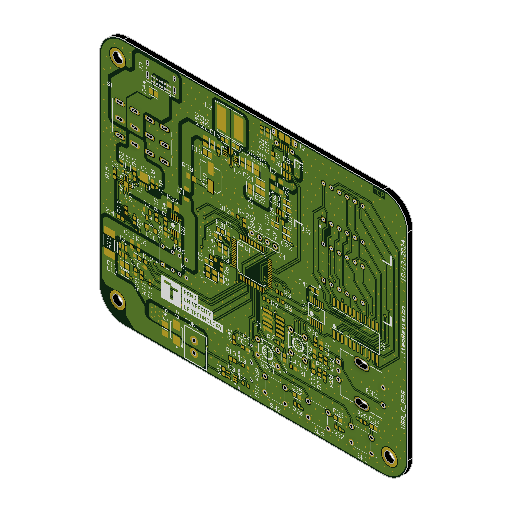
# Autodesk Inventor part: USB_C_PD_PPS_sink_BOARD
Saved by Autodesk Inventor 2025 (Build 290162000, 162)
## iProperties
Created: 2024-12-02
Part Number: USB_C_PD_PPS_sink_BOARD
Material: Generic
Document SubType Name: Modeling
Designer: Jan Mareš
Density: 1 g/cm^3
Appearance: BoardColor
Author: Jan Mareš
Autodesk Inventor part; units mm, degrees
ref_plane "YZ Plane" through (0, 0, 0) normal (1, 0, 0) x (0, 1, 0)
ref_plane "XZ Plane" through (0, 0, 0) normal (0, 1, 0) x (-1, 0, 0)
ref_plane "BoardFrontPlane" through (0, 0, 0) normal (0, 0, 1) x (1, 0, 0)
sketch "Sketch1" plane through (0, 0, 0) normal (0, 0, 1) x (1, 0, 0)
  arc A0 (0.0064, 8.0063) -> (8.0063, 0.0064) centre (8.0063, 8.0063) ccw
  line L0 (0.0064, 8.0063) -> (0.0064, 72.0063)
  arc A1 (8.0063, 80.0064) -> (0.0064, 72.0063) centre (8.0063, 72.0064) ccw
  line L1 (8.0063, 80.0064) -> (92.0063, 80.0064)
  arc A2 (100.0064, 72.0063) -> (92.0063, 80.0064) centre (92.0063, 72.0063) ccw
  line L2 (100.0064, 72.0063) -> (100.0064, 8.0063)
  arc A3 (92.0063, 0.0064) -> (100.0064, 8.0063) centre (92.0064, 8.0063) ccw
  line L3 (92.0063, 0.0064) -> (8.0063, 0.0064)
  constraints: 8 end point, 8 point on circle, 4 centre point
extrude "BoardOutline" add sketch "Sketch1" along normal blind 1.586
sketch "Sketch14" plane through (0, 0, 1.586) normal (0, 0, 1) x (1, 0, 0)
  point P0 (66.625, 25.884)
hole "S2-4" at (66.625, 25.884, 1.586) direction (0, 0, -1) diameter 1 end through all
sketch "Sketch15" plane through (0, 0, 1.586) normal (0, 0, 1) x (1, 0, 0)
  point P0 (66.625, 19.384)
hole "S2-3" at (66.625, 19.384, 1.586) direction (0, 0, -1) diameter 1 end through all
sketch "Sketch16" plane through (0, 0, 1.586) normal (0, 0, 1) x (1, 0, 0)
  point P0 (62.125, 25.884)
hole "S2-2" at (62.125, 25.884, 1.586) direction (0, 0, -1) diameter 1 end through all
sketch "Sketch17" plane through (0, 0, 1.586) normal (0, 0, 1) x (1, 0, 0)
  point P0 (62.125, 19.384)
hole "S2-1" at (62.125, 19.384, 1.586) direction (0, 0, -1) diameter 1 end through all
sketch "Sketch18" plane through (0, 0, 1.586) normal (0, 0, 1) x (1, 0, 0)
  point P0 (57.03, 46.534)
hole "J4-1" at (57.03, 46.534, 1.586) direction (0, 0, -1) diameter 1.02 end through all
sketch "Sketch19" plane through (0, 0, 1.586) normal (0, 0, 1) x (1, 0, 0)
  point P0 (49.41, 46.534)
hole "J4-4" at (49.41, 46.534, 1.586) direction (0, 0, -1) diameter 1.02 end through all
sketch "Sketch20" plane through (0, 0, 1.586) normal (0, 0, 1) x (1, 0, 0)
  point P0 (51.95, 46.534)
hole "J4-3" at (51.95, 46.534, 1.586) direction (0, 0, -1) diameter 1.02 end through all
sketch "Sketch21" plane through (0, 0, 1.586) normal (0, 0, 1) x (1, 0, 0)
  point P0 (54.49, 46.534)
hole "J4-2" at (54.49, 46.534, 1.586) direction (0, 0, -1) diameter 1.02 end through all
sketch "Sketch34" plane through (0, 0, 1.586) normal (0, 0, 1) x (1, 0, 0)
  line L0 (12.13, 57.134) -> (10.86, 57.134) construction
  line L1 (12.13, 57.564) -> (10.86, 57.564)
  line L2 (10.86, 56.704) -> (12.13, 56.704)
  arc A0 (12.13, 56.704) -> (12.13, 57.564) centre (12.13, 57.134) ccw
  arc A1 (10.86, 57.564) -> (10.86, 56.704) centre (10.86, 57.134) ccw
  point P0 (11.495, 57.134)
  constraints: 8 end point, 4 point on circle, 4 tangent, 2 centre point, 1 midpoint, 1 parallel
extrude "S1-5" cut sketch "Sketch34" against normal through all
sketch "Sketch35" plane through (0, 0, 1.586) normal (0, 0, 1) x (1, 0, 0)
  line L0 (7.3, 57.134) -> (6.03, 57.134) construction
  line L1 (7.3, 57.564) -> (6.03, 57.564)
  line L2 (6.03, 56.704) -> (7.3, 56.704)
  arc A0 (7.3, 56.704) -> (7.3, 57.564) centre (7.3, 57.134) ccw
  arc A1 (6.03, 57.564) -> (6.03, 56.704) centre (6.03, 57.134) ccw
  point P0 (6.665, 57.134)
  constraints: 8 end point, 4 point on circle, 4 tangent, 2 centre point, 1 midpoint, 1 parallel
extrude "S1-2" cut sketch "Sketch35" against normal through all
sketch "Sketch36" plane through (0, 0, 1.586) normal (0, 0, 1) x (1, 0, 0)
  line L0 (21.79, 57.134) -> (20.52, 57.134) construction
  line L1 (21.79, 57.564) -> (20.52, 57.564)
  line L2 (20.52, 56.704) -> (21.79, 56.704)
  arc A0 (21.79, 56.704) -> (21.79, 57.564) centre (21.79, 57.134) ccw
  arc A1 (20.52, 57.564) -> (20.52, 56.704) centre (20.52, 57.134) ccw
  point P0 (21.155, 57.134)
  constraints: 8 end point, 4 point on circle, 4 tangent, 2 centre point, 1 midpoint, 1 parallel
extrude "S1-11" cut sketch "Sketch36" against normal through all
sketch "Sketch37" plane through (0, 0, 1.586) normal (0, 0, 1) x (1, 0, 0)
  line L0 (16.96, 57.134) -> (15.69, 57.134) construction
  line L1 (16.96, 57.564) -> (15.69, 57.564)
  line L2 (15.69, 56.704) -> (16.96, 56.704)
  arc A0 (16.96, 56.704) -> (16.96, 57.564) centre (16.96, 57.134) ccw
  arc A1 (15.69, 57.564) -> (15.69, 56.704) centre (15.69, 57.134) ccw
  point P0 (16.325, 57.134)
  constraints: 8 end point, 4 point on circle, 4 tangent, 2 centre point, 1 midpoint, 1 parallel
extrude "S1-8" cut sketch "Sketch37" against normal through all
sketch "Sketch38" plane through (0, 0, 1.586) normal (0, 0, 1) x (1, 0, 0)
  line L0 (12.13, 61.834) -> (10.86, 61.834) construction
  line L1 (12.13, 62.264) -> (10.86, 62.264)
  line L2 (10.86, 61.404) -> (12.13, 61.404)
  arc A0 (12.13, 61.404) -> (12.13, 62.264) centre (12.13, 61.834) ccw
  arc A1 (10.86, 62.264) -> (10.86, 61.404) centre (10.86, 61.834) ccw
  point P0 (11.495, 61.834)
  constraints: 8 end point, 4 point on circle, 4 tangent, 2 centre point, 1 midpoint, 1 parallel
extrude "S1-6" cut sketch "Sketch38" against normal through all
sketch "Sketch39" plane through (0, 0, 1.586) normal (0, 0, 1) x (1, 0, 0)
  line L0 (7.3, 61.834) -> (6.03, 61.834) construction
  line L1 (7.3, 62.264) -> (6.03, 62.264)
  line L2 (6.03, 61.404) -> (7.3, 61.404)
  arc A0 (7.3, 61.404) -> (7.3, 62.264) centre (7.3, 61.834) ccw
  arc A1 (6.03, 62.264) -> (6.03, 61.404) centre (6.03, 61.834) ccw
  point P0 (6.665, 61.834)
  constraints: 8 end point, 4 point on circle, 4 tangent, 2 centre point, 1 midpoint, 1 parallel
extrude "S1-3" cut sketch "Sketch39" against normal through all
sketch "Sketch40" plane through (0, 0, 1.586) normal (0, 0, 1) x (1, 0, 0)
  line L0 (21.79, 61.834) -> (20.52, 61.834) construction
  line L1 (21.79, 62.264) -> (20.52, 62.264)
  line L2 (20.52, 61.404) -> (21.79, 61.404)
  arc A0 (21.79, 61.404) -> (21.79, 62.264) centre (21.79, 61.834) ccw
  arc A1 (20.52, 62.264) -> (20.52, 61.404) centre (20.52, 61.834) ccw
  point P0 (21.155, 61.834)
  constraints: 8 end point, 4 point on circle, 4 tangent, 2 centre point, 1 midpoint, 1 parallel
extrude "S1-12" cut sketch "Sketch40" against normal through all
sketch "Sketch41" plane through (0, 0, 1.586) normal (0, 0, 1) x (1, 0, 0)
  line L0 (16.96, 61.834) -> (15.69, 61.834) construction
  line L1 (16.96, 62.264) -> (15.69, 62.264)
  line L2 (15.69, 61.404) -> (16.96, 61.404)
  arc A0 (16.96, 61.404) -> (16.96, 62.264) centre (16.96, 61.834) ccw
  arc A1 (15.69, 62.264) -> (15.69, 61.404) centre (15.69, 61.834) ccw
  point P0 (16.325, 61.834)
  constraints: 8 end point, 4 point on circle, 4 tangent, 2 centre point, 1 midpoint, 1 parallel
extrude "S1-9" cut sketch "Sketch41" against normal through all
sketch "Sketch42" plane through (0, 0, 1.586) normal (0, 0, 1) x (1, 0, 0)
  line L0 (16.96, 52.434) -> (15.69, 52.434) construction
  line L1 (16.96, 52.864) -> (15.69, 52.864)
  line L2 (15.69, 52.004) -> (16.96, 52.004)
  arc A0 (16.96, 52.004) -> (16.96, 52.864) centre (16.96, 52.434) ccw
  arc A1 (15.69, 52.864) -> (15.69, 52.004) centre (15.69, 52.434) ccw
  point P0 (16.325, 52.434)
  constraints: 8 end point, 4 point on circle, 4 tangent, 2 centre point, 1 midpoint, 1 parallel
extrude "S1-7" cut sketch "Sketch42" against normal through all
sketch "Sketch43" plane through (0, 0, 1.586) normal (0, 0, 1) x (1, 0, 0)
  line L0 (21.79, 52.434) -> (20.52, 52.434) construction
  line L1 (21.79, 52.864) -> (20.52, 52.864)
  line L2 (20.52, 52.004) -> (21.79, 52.004)
  arc A0 (21.79, 52.004) -> (21.79, 52.864) centre (21.79, 52.434) ccw
  arc A1 (20.52, 52.864) -> (20.52, 52.004) centre (20.52, 52.434) ccw
  point P0 (21.155, 52.434)
  constraints: 8 end point, 4 point on circle, 4 tangent, 2 centre point, 1 midpoint, 1 parallel
extrude "S1-10" cut sketch "Sketch43" against normal through all
sketch "Sketch44" plane through (0, 0, 1.586) normal (0, 0, 1) x (1, 0, 0)
  line L0 (7.3, 52.434) -> (6.03, 52.434) construction
  line L1 (7.3, 52.864) -> (6.03, 52.864)
  line L2 (6.03, 52.004) -> (7.3, 52.004)
  arc A0 (7.3, 52.004) -> (7.3, 52.864) centre (7.3, 52.434) ccw
  arc A1 (6.03, 52.864) -> (6.03, 52.004) centre (6.03, 52.434) ccw
  point P0 (6.665, 52.434)
  constraints: 8 end point, 4 point on circle, 4 tangent, 2 centre point, 1 midpoint, 1 parallel
extrude "S1-1" cut sketch "Sketch44" against normal through all
sketch "Sketch45" plane through (0, 0, 1.586) normal (0, 0, 1) x (1, 0, 0)
  line L0 (12.13, 52.434) -> (10.86, 52.434) construction
  line L1 (12.13, 52.864) -> (10.86, 52.864)
  line L2 (10.86, 52.004) -> (12.13, 52.004)
  arc A0 (12.13, 52.004) -> (12.13, 52.864) centre (12.13, 52.434) ccw
  arc A1 (10.86, 52.864) -> (10.86, 52.004) centre (10.86, 52.434) ccw
  point P0 (11.495, 52.434)
  constraints: 8 end point, 4 point on circle, 4 tangent, 2 centre point, 1 midpoint, 1 parallel
extrude "S1-4" cut sketch "Sketch45" against normal through all
sketch "Sketch46" plane through (0, 0, 1.586) normal (0, 0, 1) x (1, 0, 0)
  point P0 (20.625, 28.409)
hole "K1-8" at (20.625, 28.409, 1.586) direction (0, 0, -1) diameter 0.8 end through all
sketch "Sketch47" plane through (0, 0, 1.586) normal (0, 0, 1) x (1, 0, 0)
  point P0 (23.825, 28.409)
hole "K1-7" at (23.825, 28.409, 1.586) direction (0, 0, -1) diameter 0.8 end through all
sketch "Sketch48" plane through (0, 0, 1.586) normal (0, 0, 1) x (1, 0, 0)
  point P0 (26.025, 28.409)
hole "K1-6" at (26.025, 28.409, 1.586) direction (0, 0, -1) diameter 0.8 end through all
sketch "Sketch49" plane through (0, 0, 1.586) normal (0, 0, 1) x (1, 0, 0)
  point P0 (28.225, 28.409)
hole "K1-5" at (28.225, 28.409, 1.586) direction (0, 0, -1) diameter 0.8 end through all
sketch "Sketch50" plane through (0, 0, 1.586) normal (0, 0, 1) x (1, 0, 0)
  point P0 (28.225, 23.329)
hole "K1-4" at (28.225, 23.329, 1.586) direction (0, 0, -1) diameter 0.8 end through all
sketch "Sketch51" plane through (0, 0, 1.586) normal (0, 0, 1) x (1, 0, 0)
  point P0 (26.025, 23.329)
hole "K1-3" at (26.025, 23.329, 1.586) direction (0, 0, -1) diameter 0.8 end through all
sketch "Sketch52" plane through (0, 0, 1.586) normal (0, 0, 1) x (1, 0, 0)
  point P0 (23.825, 23.329)
hole "K1-2" at (23.825, 23.329, 1.586) direction (0, 0, -1) diameter 0.8 end through all
sketch "Sketch53" plane through (0, 0, 1.586) normal (0, 0, 1) x (1, 0, 0)
  point P0 (20.625, 23.329)
hole "K1-1" at (20.625, 23.329, 1.586) direction (0, 0, -1) diameter 0.8 end through all
sketch "Sketch54" plane through (0, 0, 1.586) normal (0, 0, 1) x (1, 0, 0)
  line L0 (24.325, 77.744) -> (24.325, 76.944) construction
  line L1 (24.025, 77.744) -> (24.025, 76.944)
  line L2 (24.625, 76.944) -> (24.625, 77.744)
  arc A0 (24.625, 77.744) -> (24.025, 77.744) centre (24.325, 77.744) ccw
  arc A1 (24.025, 76.944) -> (24.625, 76.944) centre (24.325, 76.944) ccw
  point P0 (24.325, 77.344)
  constraints: 8 end point, 4 point on circle, 4 tangent, 2 centre point, 1 midpoint, 1 parallel
extrude "J3-3" cut sketch "Sketch54" against normal through all
sketch "Sketch55" plane through (0, 0, 1.586) normal (0, 0, 1) x (1, 0, 0)
  line L0 (15.675, 77.744) -> (15.675, 76.944) construction
  line L1 (15.375, 77.744) -> (15.375, 76.944)
  line L2 (15.975, 76.944) -> (15.975, 77.744)
  arc A0 (15.975, 77.744) -> (15.375, 77.744) centre (15.675, 77.744) ccw
  arc A1 (15.375, 76.944) -> (15.975, 76.944) centre (15.675, 76.944) ccw
  point P0 (15.675, 77.344)
  constraints: 8 end point, 4 point on circle, 4 tangent, 2 centre point, 1 midpoint, 1 parallel
extrude "J3-4" cut sketch "Sketch55" against normal through all
sketch "Sketch56" plane through (0, 0, 1.586) normal (0, 0, 1) x (1, 0, 0)
  line L0 (24.325, 74.714) -> (24.325, 73.214) construction
  line L1 (24.025, 74.714) -> (24.025, 73.214)
  line L2 (24.625, 73.214) -> (24.625, 74.714)
  arc A0 (24.625, 74.714) -> (24.025, 74.714) centre (24.325, 74.714) ccw
  arc A1 (24.025, 73.214) -> (24.625, 73.214) centre (24.325, 73.214) ccw
  point P0 (24.325, 73.964)
  constraints: 8 end point, 4 point on circle, 4 tangent, 2 centre point, 1 midpoint, 1 parallel
extrude "J3-1" cut sketch "Sketch56" against normal through all
sketch "Sketch57" plane through (0, 0, 1.586) normal (0, 0, 1) x (1, 0, 0)
  line L0 (15.675, 74.714) -> (15.675, 73.214) construction
  line L1 (15.375, 74.714) -> (15.375, 73.214)
  line L2 (15.975, 73.214) -> (15.975, 74.714)
  arc A0 (15.975, 74.714) -> (15.375, 74.714) centre (15.675, 74.714) ccw
  arc A1 (15.375, 73.214) -> (15.975, 73.214) centre (15.675, 73.214) ccw
  point P0 (15.675, 73.964)
  constraints: 8 end point, 4 point on circle, 4 tangent, 2 centre point, 1 midpoint, 1 parallel
extrude "J3-2" cut sketch "Sketch57" against normal through all
sketch "Sketch58" plane through (0, 0, 1.586) normal (0, 0, 1) x (1, 0, 0)
  point P0 (22.975, 72.984)
hole "J3-A1" at (22.975, 72.984, 1.586) direction (0, 0, -1) diameter 0.4 end through all
sketch "Sketch59" plane through (0, 0, 1.586) normal (0, 0, 1) x (1, 0, 0)
  point P0 (22.125, 72.984)
hole "J3-A4" at (22.125, 72.984, 1.586) direction (0, 0, -1) diameter 0.4 end through all
sketch "Sketch60" plane through (0, 0, 1.586) normal (0, 0, 1) x (1, 0, 0)
  point P0 (21.275, 72.984)
hole "J3-A5" at (21.275, 72.984, 1.586) direction (0, 0, -1) diameter 0.4 end through all
sketch "Sketch61" plane through (0, 0, 1.586) normal (0, 0, 1) x (1, 0, 0)
  point P0 (20.425, 72.984)
hole "J3-A6" at (20.425, 72.984, 1.586) direction (0, 0, -1) diameter 0.4 end through all
sketch "Sketch62" plane through (0, 0, 1.586) normal (0, 0, 1) x (1, 0, 0)
  point P0 (19.575, 72.984)
hole "J3-A7" at (19.575, 72.984, 1.586) direction (0, 0, -1) diameter 0.4 end through all
sketch "Sketch63" plane through (0, 0, 1.586) normal (0, 0, 1) x (1, 0, 0)
  point P0 (18.725, 72.984)
hole "J3-A8" at (18.725, 72.984, 1.586) direction (0, 0, -1) diameter 0.4 end through all
sketch "Sketch64" plane through (0, 0, 1.586) normal (0, 0, 1) x (1, 0, 0)
  point P0 (17.875, 72.984)
hole "J3-A9" at (17.875, 72.984, 1.586) direction (0, 0, -1) diameter 0.4 end through all
sketch "Sketch65" plane through (0, 0, 1.586) normal (0, 0, 1) x (1, 0, 0)
  point P0 (17.025, 72.984)
hole "J3-A12" at (17.025, 72.984, 1.586) direction (0, 0, -1) diameter 0.4 end through all
sketch "Sketch66" plane through (0, 0, 1.586) normal (0, 0, 1) x (1, 0, 0)
  point P0 (17.025, 74.334)
hole "J3-B1" at (17.025, 74.334, 1.586) direction (0, 0, -1) diameter 0.4 end through all
sketch "Sketch67" plane through (0, 0, 1.586) normal (0, 0, 1) x (1, 0, 0)
  point P0 (17.875, 74.334)
hole "J3-B4" at (17.875, 74.334, 1.586) direction (0, 0, -1) diameter 0.4 end through all
sketch "Sketch68" plane through (0, 0, 1.586) normal (0, 0, 1) x (1, 0, 0)
  point P0 (18.725, 74.334)
hole "J3-B5" at (18.725, 74.334, 1.586) direction (0, 0, -1) diameter 0.4 end through all
sketch "Sketch69" plane through (0, 0, 1.586) normal (0, 0, 1) x (1, 0, 0)
  point P0 (19.575, 74.334)
hole "J3-B6" at (19.575, 74.334, 1.586) direction (0, 0, -1) diameter 0.4 end through all
sketch "Sketch70" plane through (0, 0, 1.586) normal (0, 0, 1) x (1, 0, 0)
  point P0 (20.425, 74.334)
hole "J3-B7" at (20.425, 74.334, 1.586) direction (0, 0, -1) diameter 0.4 end through all
sketch "Sketch71" plane through (0, 0, 1.586) normal (0, 0, 1) x (1, 0, 0)
  point P0 (21.275, 74.334)
hole "J3-B8" at (21.275, 74.334, 1.586) direction (0, 0, -1) diameter 0.4 end through all
sketch "Sketch72" plane through (0, 0, 1.586) normal (0, 0, 1) x (1, 0, 0)
  point P0 (22.125, 74.334)
hole "J3-B9" at (22.125, 74.334, 1.586) direction (0, 0, -1) diameter 0.4 end through all
sketch "Sketch73" plane through (0, 0, 1.586) normal (0, 0, 1) x (1, 0, 0)
  point P0 (22.975, 74.334)
hole "J3-B12" at (22.975, 74.334, 1.586) direction (0, 0, -1) diameter 0.4 end through all
sketch "Sketch74" plane through (0, 0, 1.586) normal (0, 0, 1) x (1, 0, 0)
  point P0 (57.5, 75.809)
hole "J2-7" at (57.5, 75.809, 1.586) direction (0, 0, -1) diameter 0.85 end through all
sketch "Sketch75" plane through (0, 0, 1.586) normal (0, 0, 1) x (1, 0, 0)
  point P0 (62.5, 75.809)
hole "J2-6" at (62.5, 75.809, 1.586) direction (0, 0, -1) diameter 0.85 end through all
sketch "Sketch76" plane through (0, 0, 1.586) normal (0, 0, 1) x (1, 0, 0)
  line L0 (56.5, 78.859) -> (56.5, 78.159) construction
  line L1 (56.2, 78.859) -> (56.2, 78.159)
  line L2 (56.8, 78.159) -> (56.8, 78.859)
  arc A0 (56.8, 78.859) -> (56.2, 78.859) centre (56.5, 78.859) ccw
  arc A1 (56.2, 78.159) -> (56.8, 78.159) centre (56.5, 78.159) ccw
  point P0 (56.5, 78.509)
  constraints: 8 end point, 4 point on circle, 4 tangent, 2 centre point, 1 midpoint, 1 parallel
extrude "J2-11" cut sketch "Sketch76" against normal through all
sketch "Sketch77" plane through (0, 0, 1.586) normal (0, 0, 1) x (1, 0, 0)
  line L0 (63.5, 78.859) -> (63.5, 78.159) construction
  line L1 (63.2, 78.859) -> (63.2, 78.159)
  line L2 (63.8, 78.159) -> (63.8, 78.859)
  arc A0 (63.8, 78.859) -> (63.2, 78.859) centre (63.5, 78.859) ccw
  arc A1 (63.2, 78.159) -> (63.8, 78.159) centre (63.5, 78.159) ccw
  point P0 (63.5, 78.509)
  constraints: 8 end point, 4 point on circle, 4 tangent, 2 centre point, 1 midpoint, 1 parallel
extrude "J2-8" cut sketch "Sketch77" against normal through all
sketch "Sketch78" plane through (0, 0, 1.586) normal (0, 0, 1) x (1, 0, 0)
  point P0 (77.5, 24.509)
hole "ENC1-A" at (77.5, 24.509, 1.586) direction (0, 0, -1) diameter 1 end through all
sketch "Sketch79" plane through (0, 0, 1.586) normal (0, 0, 1) x (1, 0, 0)
  point P0 (77.5, 22.009)
hole "ENC1-C" at (77.5, 22.009, 1.586) direction (0, 0, -1) diameter 1 end through all
sketch "Sketch80" plane through (0, 0, 1.586) normal (0, 0, 1) x (1, 0, 0)
  point P0 (77.5, 19.509)
hole "ENC1-B" at (77.5, 19.509, 1.586) direction (0, 0, -1) diameter 1 end through all
sketch "Sketch81" plane through (0, 0, 1.586) normal (0, 0, 1) x (1, 0, 0)
  line L0 (86, 27.609) -> (84, 27.609) construction
  line L1 (86, 28.659) -> (84, 28.659)
  line L2 (84, 26.559) -> (86, 26.559)
  arc A0 (86, 26.559) -> (86, 28.659) centre (86, 27.609) ccw
  arc A1 (84, 28.659) -> (84, 26.559) centre (84, 27.609) ccw
  point P0 (85, 27.609)
  constraints: 8 end point, 4 point on circle, 4 tangent, 2 centre point, 1 midpoint, 1 parallel
extrude "ENC1-3" cut sketch "Sketch81" against normal through all
sketch "Sketch82" plane through (0, 0, 1.586) normal (0, 0, 1) x (1, 0, 0)
  line L0 (86, 16.409) -> (84, 16.409) construction
  line L1 (86, 17.459) -> (84, 17.459)
  line L2 (84, 15.359) -> (86, 15.359)
  arc A0 (86, 15.359) -> (86, 17.459) centre (86, 16.409) ccw
  arc A1 (84, 17.459) -> (84, 15.359) centre (84, 16.409) ccw
  point P0 (85, 16.409)
  constraints: 8 end point, 4 point on circle, 4 tangent, 2 centre point, 1 midpoint, 1 parallel
extrude "ENC1-4" cut sketch "Sketch82" against normal through all
sketch "Sketch83" plane through (0, 0, 1.586) normal (0, 0, 1) x (1, 0, 0)
  point P0 (92, 24.509)
hole "ENC1-1" at (92, 24.509, 1.586) direction (0, 0, -1) diameter 1 end through all
sketch "Sketch84" plane through (0, 0, 1.586) normal (0, 0, 1) x (1, 0, 0)
  point P0 (92, 19.509)
hole "ENC1-2" at (92, 19.509, 1.586) direction (0, 0, -1) diameter 1 end through all
sketch "Sketch85" plane through (0, 0, 1.586) normal (0, 0, 1) x (1, 0, 0)
  point P0 (72.65, 55.089)
hole "DS2-7" at (72.65, 55.089, 1.586) direction (0, 0, -1) diameter 0.75 end through all
sketch "Sketch86" plane through (0, 0, 1.586) normal (0, 0, 1) x (1, 0, 0)
  point P0 (75.19, 55.089)
hole "DS2-8" at (75.19, 55.089, 1.586) direction (0, 0, -1) diameter 0.75 end through all
sketch "Sketch87" plane through (0, 0, 1.586) normal (0, 0, 1) x (1, 0, 0)
  point P0 (77.73, 55.089)
hole "DS2-9" at (77.73, 55.089, 1.586) direction (0, 0, -1) diameter 0.75 end through all
sketch "Sketch88" plane through (0, 0, 1.586) normal (0, 0, 1) x (1, 0, 0)
  point P0 (80.27, 55.089)
hole "DS2-10" at (80.27, 55.089, 1.586) direction (0, 0, -1) diameter 0.75 end through all
sketch "Sketch89" plane through (0, 0, 1.586) normal (0, 0, 1) x (1, 0, 0)
  point P0 (82.81, 55.089)
hole "DS2-11" at (82.81, 55.089, 1.586) direction (0, 0, -1) diameter 0.75 end through all
sketch "Sketch90" plane through (0, 0, 1.586) normal (0, 0, 1) x (1, 0, 0)
  point P0 (85.35, 55.089)
hole "DS2-12" at (85.35, 55.089, 1.586) direction (0, 0, -1) diameter 0.75 end through all
sketch "Sketch91" plane through (0, 0, 1.586) normal (0, 0, 1) x (1, 0, 0)
  point P0 (72.65, 44.929)
hole "DS2-1" at (72.65, 44.929, 1.586) direction (0, 0, -1) diameter 0.75 end through all
sketch "Sketch92" plane through (0, 0, 1.586) normal (0, 0, 1) x (1, 0, 0)
  point P0 (75.19, 44.929)
hole "DS2-2" at (75.19, 44.929, 1.586) direction (0, 0, -1) diameter 0.75 end through all
sketch "Sketch93" plane through (0, 0, 1.586) normal (0, 0, 1) x (1, 0, 0)
  point P0 (77.73, 44.929)
hole "DS2-3" at (77.73, 44.929, 1.586) direction (0, 0, -1) diameter 0.75 end through all
sketch "Sketch94" plane through (0, 0, 1.586) normal (0, 0, 1) x (1, 0, 0)
  point P0 (80.27, 44.929)
hole "DS2-4" at (80.27, 44.929, 1.586) direction (0, 0, -1) diameter 0.75 end through all
sketch "Sketch95" plane through (0, 0, 1.586) normal (0, 0, 1) x (1, 0, 0)
  point P0 (82.81, 44.929)
hole "DS2-5" at (82.81, 44.929, 1.586) direction (0, 0, -1) diameter 0.75 end through all
sketch "Sketch96" plane through (0, 0, 1.586) normal (0, 0, 1) x (1, 0, 0)
  point P0 (85.35, 44.929)
hole "DS2-6" at (85.35, 44.929, 1.586) direction (0, 0, -1) diameter 0.75 end through all
sketch "Sketch97" plane through (0, 0, 1.586) normal (0, 0, 1) x (1, 0, 0)
  point P0 (72.65, 72.089)
hole "DS1-7" at (72.65, 72.089, 1.586) direction (0, 0, -1) diameter 0.75 end through all
sketch "Sketch98" plane through (0, 0, 1.586) normal (0, 0, 1) x (1, 0, 0)
  point P0 (75.19, 72.089)
hole "DS1-8" at (75.19, 72.089, 1.586) direction (0, 0, -1) diameter 0.75 end through all
sketch "Sketch99" plane through (0, 0, 1.586) normal (0, 0, 1) x (1, 0, 0)
  point P0 (77.73, 72.089)
hole "DS1-9" at (77.73, 72.089, 1.586) direction (0, 0, -1) diameter 0.75 end through all
sketch "Sketch100" plane through (0, 0, 1.586) normal (0, 0, 1) x (1, 0, 0)
  point P0 (80.27, 72.089)
hole "DS1-10" at (80.27, 72.089, 1.586) direction (0, 0, -1) diameter 0.75 end through all
sketch "Sketch101" plane through (0, 0, 1.586) normal (0, 0, 1) x (1, 0, 0)
  point P0 (82.81, 72.089)
hole "DS1-11" at (82.81, 72.089, 1.586) direction (0, 0, -1) diameter 0.75 end through all
sketch "Sketch102" plane through (0, 0, 1.586) normal (0, 0, 1) x (1, 0, 0)
  point P0 (85.35, 72.089)
hole "DS1-12" at (85.35, 72.089, 1.586) direction (0, 0, -1) diameter 0.75 end through all
sketch "Sketch103" plane through (0, 0, 1.586) normal (0, 0, 1) x (1, 0, 0)
  point P0 (72.65, 61.929)
hole "DS1-1" at (72.65, 61.929, 1.586) direction (0, 0, -1) diameter 0.75 end through all
sketch "Sketch104" plane through (0, 0, 1.586) normal (0, 0, 1) x (1, 0, 0)
  point P0 (75.19, 61.929)
hole "DS1-2" at (75.19, 61.929, 1.586) direction (0, 0, -1) diameter 0.75 end through all
sketch "Sketch105" plane through (0, 0, 1.586) normal (0, 0, 1) x (1, 0, 0)
  point P0 (77.73, 61.929)
hole "DS1-3" at (77.73, 61.929, 1.586) direction (0, 0, -1) diameter 0.75 end through all
sketch "Sketch106" plane through (0, 0, 1.586) normal (0, 0, 1) x (1, 0, 0)
  point P0 (80.27, 61.929)
hole "DS1-4" at (80.27, 61.929, 1.586) direction (0, 0, -1) diameter 0.75 end through all
sketch "Sketch107" plane through (0, 0, 1.586) normal (0, 0, 1) x (1, 0, 0)
  point P0 (82.81, 61.929)
hole "DS1-5" at (82.81, 61.929, 1.586) direction (0, 0, -1) diameter 0.75 end through all
sketch "Sketch108" plane through (0, 0, 1.586) normal (0, 0, 1) x (1, 0, 0)
  point P0 (85.35, 61.929)
hole "DS1-6" at (85.35, 61.929, 1.586) direction (0, 0, -1) diameter 0.75 end through all
sketch "Sketch111" plane through (0, 0, 1.586) normal (0, 0, 1) x (1, 0, 0)
  point P0 (94, 6.009)
hole "Free-MH_UFFYUCRS" at (94, 6.009, 1.586) direction (0, 0, -1) diameter 3.2 end through all
sketch "Sketch112" plane through (0, 0, 1.586) normal (0, 0, 1) x (1, 0, 0)
  point P0 (6, 6.009)
hole "Free-MH_NTYALDTJ" at (6, 6.009, 1.586) direction (0, 0, -1) diameter 3.2 end through all
sketch "Sketch113" plane through (0, 0, 1.586) normal (0, 0, 1) x (1, 0, 0)
  point P0 (6, 74.009)
hole "Free-MH_SGBJWQGS" at (6, 74.009, 1.586) direction (0, 0, -1) diameter 3.2 end through all
sketch "Sketch115" plane through (0, 0, 1.586) normal (0, 0, 1) x (1, 0, 0)
  line L0 (88.775, 12.009) -> (32.6, 12.009)
  line L1 (32.6, 12.009) -> (32.6, 0.509)
  line L2 (32.6, 0.509) -> (88.775, 0.509)
  line L3 (88.775, 0.509) -> (88.775, 12.009)
  constraints: 8 end point
surface extrude "UI_BTNs" sketch "Sketch115" along normal blind 0.0508 shown yes curves L0 L1 L2 L3
sketch "Sketch116" plane through (0, 0, 1.586) normal (0, 0, 1) x (1, 0, 0)
  line L0 (27.15, 49.757) -> (54.875, 49.757)
  line L1 (54.875, 49.757) -> (54.875, 81.634)
  line L2 (54.875, 81.634) -> (27.15, 81.634)
  line L3 (27.15, 81.634) -> (27.15, 49.757)
  constraints: 8 end point
surface extrude "U_Buck_boost" sketch "Sketch116" along normal blind 0.0508 shown yes curves L0 L1 L2 L3
sketch "Sketch117" plane through (0, 0, 1.586) normal (0, 0, 1) x (1, 0, 0)
  line L0 (30.15, 23.087) -> (62.6, 23.087)
  line L1 (62.6, 23.087) -> (62.6, 47.921)
  line L2 (62.6, 47.921) -> (30.15, 47.921)
  line L3 (30.15, 47.921) -> (30.15, 23.087)
  constraints: 8 end point
surface extrude "MCU" sketch "Sketch117" along normal blind 0.0508 shown yes curves L0 L1 L2 L3
sketch "Sketch118" plane through (0, 0, 1.586) normal (0, 0, 1) x (1, 0, 0)
  line L0 (20.354, 28.583) -> (2.704, 28.583)
  line L1 (2.704, 28.583) -> (2.704, 13.3694)
  line L2 (2.704, 13.3694) -> (20.354, 13.3694)
  line L3 (20.354, 13.3694) -> (20.354, 28.583)
  constraints: 8 end point
surface extrude "LOAD_SENSE" sketch "Sketch118" along normal blind 0.0508 shown yes curves L0 L1 L2 L3
sketch "Sketch119" plane through (0, 0, 1.586) normal (0, 0, 1) x (1, 0, 0)
  line L0 (3.375, 32.034) -> (16.7, 32.034)
  line L1 (16.7, 32.034) -> (16.7, 46.759)
  line L2 (16.7, 46.759) -> (3.375, 46.759)
  line L3 (3.375, 46.759) -> (3.375, 32.034)
  constraints: 8 end point
surface extrude "Protection" sketch "Sketch119" along normal blind 0.0508 shown yes curves L0 L1 L2 L3
sketch "Sketch120" plane through (0, 0, 1.586) normal (0, 0, 1) x (1, 0, 0)
  line L0 (54.925, 67.061) -> (67.725, 67.061)
  line L1 (67.725, 67.061) -> (67.725, 80.086)
  line L2 (67.725, 80.086) -> (54.925, 80.086)
  line L3 (54.925, 80.086) -> (54.925, 67.061)
  constraints: 8 end point
surface extrude "USB_B" sketch "Sketch120" along normal blind 0.0508 shown yes curves L0 L1 L2 L3
sketch "Sketch121" plane through (0, 0, 1.586) normal (0, 0, 1) x (1, 0, 0)
  line L0 (55.034, 63.075) -> (55.034, 50.225)
  line L1 (55.034, 50.225) -> (62.434, 50.225)
  line L2 (62.434, 50.225) -> (62.434, 63.075)
  line L3 (62.434, 63.075) -> (55.034, 63.075)
  constraints: 8 end point
surface extrude "LDO" sketch "Sketch121" along normal blind 0.0508 shown yes curves L0 L1 L2 L3
sketch "Sketch122" plane through (0, 0, 1.586) normal (0, 0, 1) x (1, 0, 0)
  line L0 (68.488, 27.133) -> (68.488, 12.333)
  line L1 (68.488, 12.333) -> (92.888, 12.333)
  line L2 (92.888, 12.333) -> (92.888, 27.133)
  line L3 (92.888, 27.133) -> (68.488, 27.133)
  constraints: 8 end point
surface extrude "Encoder" sketch "Sketch122" along normal blind 0.0508 shown yes curves L0 L1 L2 L3
sketch "Sketch123" plane through (0, 0, 1.586) normal (0, 0, 1) x (1, 0, 0)
  line L0 (21.077, 31.904) -> (27.977, 31.904)
  line L1 (27.977, 31.904) -> (27.977, 43.304)
  line L2 (27.977, 43.304) -> (21.077, 43.304)
  line L3 (21.077, 43.304) -> (21.077, 31.904)
  constraints: 8 end point
surface extrude "OCP" sketch "Sketch123" along normal blind 0.0508 shown yes curves L0 L1 L2 L3
sketch "Sketch127" plane through (0, 0, 1.586) normal (0, 0, 1) x (1, 0, 0)
  point P0 (49.375, 5.059)
hole "LP3-TH_TUYHERHS_1" at (49.375, 5.059, 1.586) direction (0, 0, -1) diameter 0.62 end through all
sketch "Sketch129" plane through (0, 0, 1.586) normal (0, 0, 1) x (1, 0, 0)
  point P0 (45.275, 0.959)
hole "LP3-TH_AGCPFLQI_1" at (45.275, 0.959, 1.586) direction (0, 0, -1) diameter 0.62 end through all
sketch "Sketch131" plane through (0, 0, 1.586) normal (0, 0, 1) x (1, 0, 0)
  point P0 (49.375, 15.059)
hole "LP2-TH_TJIVDCAF_1" at (49.375, 15.059, 1.586) direction (0, 0, -1) diameter 0.62 end through all
sketch "Sketch133" plane through (0, 0, 1.586) normal (0, 0, 1) x (1, 0, 0)
  point P0 (45.275, 10.959)
hole "LP2-TH_ARMWKDFP_1" at (45.275, 10.959, 1.586) direction (0, 0, -1) diameter 0.62 end through all
sketch "Sketch135" plane through (0, 0, 1.586) normal (0, 0, 1) x (1, 0, 0)
  point P0 (49.375, 10.059)
hole "LP1-TH_UMCDBLLX_1" at (49.375, 10.059, 1.586) direction (0, 0, -1) diameter 0.62 end through all
sketch "Sketch137" plane through (0, 0, 1.586) normal (0, 0, 1) x (1, 0, 0)
  point P0 (45.275, 5.959)
hole "LP1-TH_UEIXYMFC_1" at (45.275, 5.959, 1.586) direction (0, 0, -1) diameter 0.62 end through all
sketch "Sketch138" plane through (0, 0, 1.586) normal (0, 0, 1) x (1, 0, 0)
  point P0 (51.325, 17.784)
hole "S3-4" at (51.325, 17.784, 1.586) direction (0, 0, -1) diameter 1 end through all
sketch "Sketch139" plane through (0, 0, 1.586) normal (0, 0, 1) x (1, 0, 0)
  point P0 (57.825, 17.784)
hole "S3-3" at (57.825, 17.784, 1.586) direction (0, 0, -1) diameter 1 end through all
sketch "Sketch140" plane through (0, 0, 1.586) normal (0, 0, 1) x (1, 0, 0)
  point P0 (51.325, 13.284)
hole "S3-2" at (51.325, 13.284, 1.586) direction (0, 0, -1) diameter 1 end through all
sketch "Sketch141" plane through (0, 0, 1.586) normal (0, 0, 1) x (1, 0, 0)
  point P0 (57.825, 13.284)
hole "S3-1" at (57.825, 13.284, 1.586) direction (0, 0, -1) diameter 1 end through all
sketch "Sketch142" plane through (0, 0, 1.586) normal (0, 0, 1) x (1, 0, 0)
  point P0 (67.7, 8.509)
hole "SW3-4" at (67.7, 8.509, 1.586) direction (0, 0, -1) diameter 1.05 end through all
sketch "Sketch143" plane through (0, 0, 1.586) normal (0, 0, 1) x (1, 0, 0)
  point P0 (74.2, 8.509)
hole "SW3-3" at (74.2, 8.509, 1.586) direction (0, 0, -1) diameter 1.05 end through all
sketch "Sketch144" plane through (0, 0, 1.586) normal (0, 0, 1) x (1, 0, 0)
  point P0 (67.7, 4.009)
hole "SW3-2" at (67.7, 4.009, 1.586) direction (0, 0, -1) diameter 1.05 end through all
sketch "Sketch145" plane through (0, 0, 1.586) normal (0, 0, 1) x (1, 0, 0)
  point P0 (74.2, 4.009)
hole "SW3-1" at (74.2, 4.009, 1.586) direction (0, 0, -1) diameter 1.05 end through all
sketch "Sketch146" plane through (0, 0, 1.586) normal (0, 0, 1) x (1, 0, 0)
  point P0 (60.2, 4.009)
hole "SW2-1" at (60.2, 4.009, 1.586) direction (0, 0, -1) diameter 1.05 end through all
sketch "Sketch147" plane through (0, 0, 1.586) normal (0, 0, 1) x (1, 0, 0)
  point P0 (53.7, 4.009)
hole "SW2-2" at (53.7, 4.009, 1.586) direction (0, 0, -1) diameter 1.05 end through all
sketch "Sketch148" plane through (0, 0, 1.586) normal (0, 0, 1) x (1, 0, 0)
  point P0 (60.2, 8.509)
hole "SW2-3" at (60.2, 8.509, 1.586) direction (0, 0, -1) diameter 1.05 end through all
sketch "Sketch149" plane through (0, 0, 1.586) normal (0, 0, 1) x (1, 0, 0)
  point P0 (53.7, 8.509)
hole "SW2-4" at (53.7, 8.509, 1.586) direction (0, 0, -1) diameter 1.05 end through all
sketch "Sketch150" plane through (0, 0, 1.586) normal (0, 0, 1) x (1, 0, 0)
  point P0 (81.7, 8.509)
hole "SW1-4" at (81.7, 8.509, 1.586) direction (0, 0, -1) diameter 1.05 end through all
sketch "Sketch151" plane through (0, 0, 1.586) normal (0, 0, 1) x (1, 0, 0)
  point P0 (88.2, 8.509)
hole "SW1-3" at (88.2, 8.509, 1.586) direction (0, 0, -1) diameter 1.05 end through all
sketch "Sketch152" plane through (0, 0, 1.586) normal (0, 0, 1) x (1, 0, 0)
  point P0 (81.7, 4.009)
hole "SW1-2" at (81.7, 4.009, 1.586) direction (0, 0, -1) diameter 1.05 end through all
sketch "Sketch153" plane through (0, 0, 1.586) normal (0, 0, 1) x (1, 0, 0)
  point P0 (88.2, 4.009)
hole "SW1-1" at (88.2, 4.009, 1.586) direction (0, 0, -1) diameter 1.05 end through all
sketch "Sketch154" plane through (0, 0, 1.586) normal (0, 0, 1) x (1, 0, 0)
  point P0 (30.75, 3.559)
hole "CON1-1" at (30.75, 3.559, 1.586) direction (0, 0, -1) diameter 1.2 end through all
sketch "Sketch155" plane through (0, 0, 1.586) normal (0, 0, 1) x (1, 0, 0)
  point P0 (30.75, 7.059)
hole "CON1-2" at (30.75, 7.059, 1.586) direction (0, 0, -1) diameter 1.2 end through all
sketch "Sketch156" plane through (0, 0, 1.586) normal (0, 0, 1) x (1, 0, 0)
  line L0 (41.4, 0.225) -> (52.125, 0.225)
  line L1 (52.125, 0.225) -> (52.125, 15.775)
  line L2 (52.125, 15.775) -> (41.4, 15.775)
  line L3 (41.4, 15.775) -> (41.4, 0.225)
  constraints: 8 end point
surface extrude "RoomDefinition" sketch "Sketch156" along normal blind 0.0508 shown yes curves L0 L1 L2 L3
sketch "img_Top" plane through (0, 0, 1.586) normal (0, 0, 1) x (1, 0, 0)
  line L0 (0.0064, 80.0064) -> (100.0064, 80.0064) construction
  line L1 (100.0064, 80.0064) -> (100.0064, -0.0038) construction
  line L2 (100.0064, -0.0038) -> (0.0064, -0.0038) construction
  line L3 (0.0064, -0.0038) -> (0.0064, 80.0064) construction
  constraints: 2 other
decal "Decal_Top"
sketch "img_Bottom" plane through (0, 0, -1.586) normal (0, 0, -1) x (1, 0, 0)
  line L0 (0.0064, -0.0064) -> (100.0064, -0.0063) construction
  line L1 (100.0064, -0.0063) -> (100.0064, -80.0165) construction
  line L2 (100.0064, -80.0165) -> (0.0064, -80.0165) construction
  line L3 (0.0064, -80.0165) -> (0.0064, -0.0064) construction
  constraints: 2 other
decal "Decal_Bottom"
body "Solid1"
body "Srf2"
body "Srf3"
body "Srf4"
body "Srf5"
body "Srf6"
body "Srf7"
body "Srf8"
body "Srf9"
body "Srf10"
body "Srf11"
